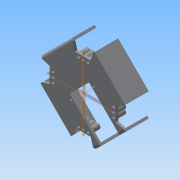
# Autodesk Inventor part: head
Saved by Autodesk Inventor 2015 (Build 190159000, 159)
## iProperties
Created: 2015-06-18
Part Number: head
Material: Générique
Document SubType Name: Modeling
Designer: Gregwar
Density: 1 g/cm^3
Appearance: Par défaut
Author: Gregwar
Autodesk Inventor part; units mm, degrees
ref_plane "YZ Plane" through (0, 0, 0) normal (1, 0, 0) x (0, 1, 0)
ref_plane "XZ Plane" through (0, 0, 0) normal (0, 1, 0) x (-1, 0, 0)
ref_plane "XY Plane" through (0, 0, 0) normal (0, 0, 1) x (1, 0, 0)
sketch "Esquisse1" plane through (0, 0, 0) normal (0, 1, 0) x (-1, 0, 0)
  line L0 (35, 35) -> (35, 14)
  line L1 (35, 14) -> (42, 10)
  line L2 (42, 10) -> (42, 0)
  line L3 (35, 35) -> (0, 0)
  line L4 (42, 0) -> (0, 0) construction
  line L5 (35, -35) -> (35, -14)
  line L6 (35, -14) -> (42, -10)
  line L7 (42, -10) -> (42, 0)
  line L8 (35, -35) -> (0, 0)
  line L9 (38.5, -12) -> (38.5, 12) construction
  circle A0 centre (38.5, 0) radius 2.15
  circle A1 centre (38.5, 6) radius 2.15
  circle A2 centre (38.5, -6) radius 2.15
  dimension "d0" = 90
  dimension "d1" = 70
  dimension "d4" = 6
  dimension "d11" = 6
  dimension "d16" = 4.3
  dimension "d17" = 20
  dimension "d18" = 4
  dimension "d19" = 7
  constraints: 20 end point, 3 centre point, 3 midpoint, 3 symmetric about line, 3 vertical, 1 horizontal, 1 parallel, 4 other
  measures "d0" angle of L3 L8
  measures "d1" distance of L0.start L5.start
  measures "d4" distance of A0.centre A1.centre
  measures "d11" distance of A0.centre A2.centre
  measures "d16" diameter of A0
  measures "d17" distance of L1.end L6.end
  measures "d18" vertical distance of L1.end L0.end
  measures "d19" distance between parallel lines of L5 L7
extrude "Extrusion1" add sketch "Esquisse1" along normal blind 3
pattern_circular "Réseau circulaire1" count 4 over 360 about axis through (0, 0, 0) along (0, 1, 0) of "Extrusion1"
ref_plane "Plan de construction2" through (0, 0, -14) normal (1, 0, 0) x (0, 0, -1)
ref_plane "Plan de construction3" through (-14, 0, 0) normal (0, 0, -1) x (-1, 0, 0)
chamfer "Chanfrein1" distance 10 angle 45 4 edges at (-35, 1.5, -35) (-35, 1.5, 35) (35, 1.5, -35) (35, 1.5, 35)
sketch "Esquisse3" plane through (0, 0, 0) normal (0, -1, 0) x (1, 0, 0)
  circle A0 centre (0, 38.5) radius 2.15 construction
  circle A1 centre (6, 38.5) radius 2.15 construction
  circle A2 centre (-6, 38.5) radius 2.15 construction
  circle A3 centre (38.5, 6) radius 2.15 construction
  circle A4 centre (38.5, -6) radius 2.15 construction
  circle A5 centre (38.5, 0) radius 2.15 construction
  circle A6 centre (6, -38.5) radius 2.15 construction
  circle A7 centre (-6, -38.5) radius 2.15 construction
  circle A8 centre (0, -38.5) radius 2.15 construction
  circle A9 centre (-38.5, -6) radius 2.15 construction
  circle A10 centre (-38.5, 6) radius 2.15 construction
  circle A11 centre (-38.5, 0) radius 2.15 construction
  line L0 (-35, 25) -> (-35, 14) construction
  line L1 (-35, 14) -> (-42, 10) construction
  line L2 (-42, 10) -> (-42, -10) construction
  line L3 (-42, -10) -> (-35, -14) construction
  line L4 (-35, -14) -> (-35, -25) construction
  line L5 (-25, -35) -> (-14, -35) construction
  line L6 (-14, -35) -> (-10, -42) construction
  line L7 (-10, -42) -> (10, -42) construction
  line L8 (10, -42) -> (14, -35) construction
  line L9 (14, -35) -> (25, -35) construction
  line L10 (35, -25) -> (35, -14) construction
  line L11 (35, -14) -> (42, -10) construction
  line L12 (42, -10) -> (42, 10) construction
  line L13 (42, 10) -> (35, 14) construction
  line L14 (35, 14) -> (35, 25) construction
  line L15 (25, 35) -> (14, 35) construction
  line L16 (14, 35) -> (10, 42) construction
  line L17 (10, 42) -> (-10, 42) construction
  line L18 (-10, 42) -> (-14, 35) construction
  line L19 (-14, 35) -> (-25, 35) construction
  line L20 (-51.72, -12.8291) -> (-12.8291, -51.72)
  line L21 (-12.8291, -51.72) -> (-10, -42)
  line L22 (-42, -10) -> (-51.72, -12.8291)
  line L23 (-35, -14) -> (-42, -10)
  line L24 (-42, -10) -> (-35, -14) projected
  line L25 (-10, -42) -> (-14, -35)
  line L26 (-14, -35) -> (-10, -42) projected
  line L27 (25, 35) -> (35, 25) projected
  line L28 (-35, 25) -> (-25, 35) projected
  line L29 (-25, -35) -> (-35, -25) projected
  line L30 (35, -25) -> (25, -35) projected
  line L31 (-14, -35) -> (-35, -14)
  point P0 (0, 0)
  dimension "d32" = 135
  dimension "d33" = 55
  constraints: 12 end point, 1 collinear, 1 equal length, 1 point on line
  measures "d32" angle of L5 L20
  measures "d33" distance of L20.start L20.end
extrude "Extrusion3" add sketch "Esquisse3" against normal blind 3
sketch "Esquisse4" plane through (-51.72, 0, -12.8291) normal (-0.7071068, 0, -0.7071068) x (-0.7071068, 0, 0.7071068)
  line L0 (0, 0) -> (-55, 0) construction
  line L1 (0, 0) -> (0, 3) construction
  line L2 (-55, 3) -> (0, 3) construction
  line L3 (-55, 0) -> (-55, 3) construction
  line L4 (0, 0) -> (-55, 0)
  line L5 (-55, 0) -> (-55, 30)
  line L6 (-55, 30) -> (0, 30)
  line L7 (0, 30) -> (0, 0)
  point P0 (-27.5, 0)
  dimension "d36" = 30
  constraints: 8 end point, 2 parallel, 1 horizontal, 1 perpendicular
  measures "d36" distance of L4.end L5.end
extrude "Extrusion4" add sketch "Esquisse4" along normal blind 3
sketch "Esquisse5" plane through (-53.8413, 0, -14.9504) normal (-0.7071068, 0, -0.7071068) x (-0.7071068, 0, 0.7071068)
  line L0 (-55, 0) -> (0, 0) construction
  line L1 (0, 0) -> (0, 30) construction
  line L2 (0, 30) -> (-55, 30) construction
  line L3 (-55, 30) -> (-55, 0) construction
  line L4 (0, 0) -> (0, 30) construction
  line L5 (0, 13.8206) -> (-55, 13.8206) construction
  circle A0 centre (-15.1412, 13.8206) radius 7.3571
  line L6 (-27.5, 0) -> (-27.5, 30) construction
  circle A1 centre (-39.8588, 13.8206) radius 7.3571
  constraints: 4 end point, 3 point on line, 2 centre point, 1 midpoint, 1 perpendicular, 1 symmetric about line, 1 other
extrude "Extrusion5" cut sketch "Esquisse5" against normal blind 1
pattern_circular "Réseau circulaire2" count 4 over 360 about axis through (0, 0, 0) along (0, -1, 0) of "Extrusion3", "Extrusion4"
fillet "Congé1" radius 3 2 edges at (-34.3959, 0, 34.3959) (34.3959, 0, -34.3959)
sketch "Esquisse6" plane through (0, 0, 0) normal (0, -1, 0) x (1, 0, 0)
  line L0 (51.72, -12.8291) -> (12.8291, -51.72) construction
  line L1 (51.72, -12.8291) -> (42, -10) construction
  line L2 (42, -10) -> (42, 10) construction
  line L3 (42, 10) -> (51.72, 12.8291) construction
  line L4 (51.72, 12.8291) -> (53.8413, 14.9504) construction
  line L5 (14.9504, 53.8413) -> (53.8413, 14.9504) construction
  line L6 (12.8291, 51.72) -> (14.9504, 53.8413) construction
  line L7 (12.8291, 51.72) -> (10, 42) construction
  line L8 (10, 42) -> (-10, 42) construction
  line L9 (-10, 42) -> (-12.8291, 51.72) construction
  line L10 (-51.72, 12.8291) -> (-12.8291, 51.72) construction
  line L11 (-51.72, 12.8291) -> (-42, 10) construction
  line L12 (-42, 10) -> (-42, -10) construction
  line L13 (-42, -10) -> (-51.72, -12.8291) construction
  line L14 (-51.72, -12.8291) -> (-53.8413, -14.9504) construction
  line L15 (-14.9504, -53.8413) -> (-53.8413, -14.9504) construction
  line L16 (-12.8291, -51.72) -> (-14.9504, -53.8413) construction
  line L17 (-12.8291, -51.72) -> (-10, -42) construction
  line L18 (-10, -42) -> (10, -42) construction
  line L19 (10, -42) -> (12.8291, -51.72) construction
  circle A0 centre (0, 38.5) radius 2.15 construction
  circle A1 centre (6, 38.5) radius 2.15 construction
  circle A2 centre (-6, 38.5) radius 2.15 construction
  circle A3 centre (38.5, 6) radius 2.15 construction
  circle A4 centre (38.5, -6) radius 2.15 construction
  circle A5 centre (38.5, 0) radius 2.15 construction
  circle A6 centre (6, -38.5) radius 2.15 construction
  circle A7 centre (-6, -38.5) radius 2.15 construction
  circle A8 centre (0, -38.5) radius 2.15 construction
  circle A9 centre (-38.5, -6) radius 2.15 construction
  circle A10 centre (-38.5, 6) radius 2.15 construction
  circle A11 centre (-38.5, 0) radius 2.15 construction
  line L20 (14.9504, -53.8413) -> (53.8413, -14.9504) construction
  line L21 (22.0215, -46.7702) -> (-16.8694, -7.8793)
  line L22 (-16.8694, -7.8793) -> (7.8793, 16.8694)
  line L23 (7.8793, 16.8694) -> (46.7702, -22.0215)
  line L24 (46.7702, -22.0215) -> (22.0215, -46.7702)
  line L25 (-16.8694, -7.8793) -> (-13.3339, -11.4149) construction
  line L26 (-13.3339, -11.4149) -> (11.4149, 13.3339) construction
  line L27 (11.4149, 13.3339) -> (7.8793, 16.8694) construction
  line L28 (-4.495, 4.495) -> (34.3959, -34.3959) construction
  line L29 (-13.3339, -11.4149) -> (-30.7818, -28.8628) construction
  circle A12 centre (-15.4552, -13.5362) radius 1.7
  circle A13 centre (13.5362, 15.4552) radius 1.7
  point P0 (0, 0)
  dimension "d48" = 35
  dimension "d49" = 55
  dimension "d54" = 35
  dimension "d69" = 5
  dimension "d70" = 3
  dimension "d71" = 3.4
  constraints: 18 end point, 4 perpendicular, 3 collinear, 3 midpoint, 3 point on line, 2 centre point, 1 parallel, 1 symmetric about line, 1 other
  measures "d48" distance of L21.end L22.end
  measures "d49" distance of L21.start L21.end
  measures "d54" distance of L25.end L26.end
  measures "d69" distance between parallel lines of L26 L22
  measures "d70" distance from line of A12.centre L21
  measures "d71" diameter of A12
extrude "Extrusion6" cut sketch "Esquisse6" against normal through all
sketch "Esquisse8" plane through (0, 3, 0) normal (0, 1, 0) x (1, 0, 0)
  circle A0 centre (-38.5, 0) radius 2.15 projected
  circle A1 centre (-38.5, -6) radius 2.15 projected
  circle A2 centre (-38.5, 6) radius 2.15 projected
  circle A3 centre (0, 38.5) radius 2.15 construction
  circle A4 centre (-6, 38.5) radius 2.15 construction
  circle A5 centre (6, 38.5) radius 2.15 construction
  circle A6 centre (38.5, 0) radius 2.15 construction
  circle A7 centre (38.5, 6) radius 2.15 construction
  circle A8 centre (38.5, -6) radius 2.15 construction
  circle A9 centre (-6, -38.5) radius 2.15 construction
  circle A10 centre (6, -38.5) radius 2.15 construction
  circle A11 centre (0, -38.5) radius 2.15 construction
  line L0 (19.9002, 44.6489) -> (12.8291, 51.72) construction
  line L1 (12.8291, 51.72) -> (10, 42) construction
  line L2 (10, 42) -> (-10, 42) construction
  line L3 (-10, 42) -> (-12.8291, 51.72) construction
  line L4 (-12.8291, 51.72) -> (-51.72, 12.8291) construction
  line L5 (-51.72, 12.8291) -> (-42, 10) construction
  line L6 (-42, 10) -> (-42, -10) construction
  line L7 (-42, -10) -> (-51.72, -12.8291) construction
  line L8 (-51.72, -12.8291) -> (-12.8291, -51.72) construction
  line L9 (-12.8291, -51.72) -> (-10, -42) construction
  line L10 (-10, -42) -> (10, -42) construction
  line L11 (10, -42) -> (12.8291, -51.72) construction
  line L12 (12.8291, -51.72) -> (51.72, -12.8291) construction
  line L13 (51.72, -12.8291) -> (42, -10) construction
  line L14 (42, -10) -> (42, 10) construction
  line L15 (42, 10) -> (51.72, 12.8291) construction
  circle A12 centre (-38.5, -6) radius 3.5
  circle A13 centre (-38.5, 0) radius 3.5
  circle A14 centre (-38.5, 6) radius 3.5
  line L16 (44.6489, 19.9002) -> (7.8793, -16.8694) projected
  line L17 (7.8793, -16.8694) -> (-16.8694, 7.8793) projected
  line L18 (-16.8694, 7.8793) -> (19.9002, 44.6489) projected
  line L19 (51.72, 12.8291) -> (44.6489, 19.9002) projected
  point P0 (0, 0)
  dimension "d91" = 6
  dimension "d96" = 7
  constraints: 3 centre point, 1 coincident, 1 vertical, 4 other
  measures "d91" distance of A12.centre A13.centre
  measures "d96" diameter of A12
extrude "Extrusion8" add sketch "Esquisse8" along normal blind 10
pattern_circular "Réseau circulaire4" count 4 over 360 about axis through (0, 0, 0) along (0, -1, 0) of "Extrusion8"
sketch "Esquisse9" plane through (53.8413, 3, -14.9504) normal (0.7071068, 0, -0.7071068) x (-0.7071068, 0, -0.7071068)
  line L0 (10, 0) -> (10, 27) construction
  line L1 (10, 27) -> (0, 27) construction
  line L2 (0, 27) -> (0, 0) construction
  line L3 (10, 0) -> (0, 0) construction
  line L4 (45, 27) -> (45, 0) construction
  line L5 (55, 0) -> (45, 0) construction
  line L6 (55, 0) -> (55, 27) construction
  line L7 (55, 27) -> (45, 27) construction
  line L8 (55, 23) -> (0, 23) construction
  line L9 (0, 0) -> (0, 27) construction
  circle A0 centre (50, 23) radius 1.7
  line L10 (27.5, 23) -> (27.5, 0) construction
  circle A1 centre (5, 23) radius 1.7
  line L11 (55, 27) -> (45, 27) construction
  line L12 (50, 27) -> (50, 23) construction
  point P0 (27.5, -3)
  dimension "d102" = 4
  dimension "d103" = 3.4
  constraints: 6 end point, 3 point on line, 2 centre point, 2 midpoint, 2 perpendicular, 1 symmetric about line, 1 vertical, 1 other
  measures "d102" distance between parallel lines of L1 L8
  measures "d103" diameter of A0
extrude "Extrusion9" cut sketch "Esquisse9" against normal blind 10
